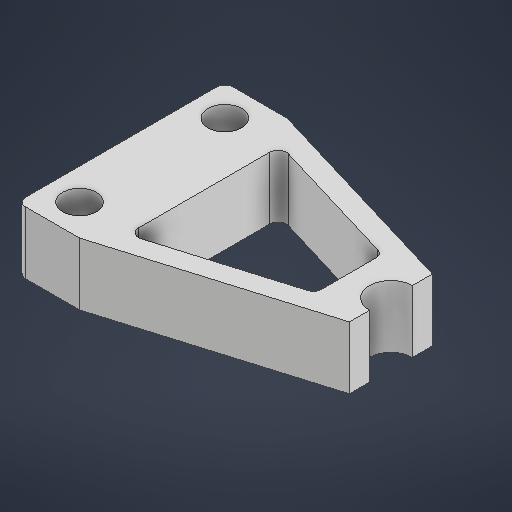
# Autodesk Inventor part: Rod_support_1
Saved by Autodesk Inventor 2026.2 (Build 302298000, 298)
## iProperties
Created: 2025-12-17
Part Number: Rod_support_1
Material: Generic
Document SubType Name: Modeling
Designer: Cobble
Density: 1 g/cm^3
Appearance: Default
Author: Cobble
Autodesk Inventor part; units mm, degrees
ref_plane "YZ Plane" through (0, 0, 0) normal (1, 0, 0) x (0, 1, 0)
ref_plane "XZ Plane" through (0, 0, 0) normal (0, 1, 0) x (-1, 0, 0)
ref_plane "XY Plane" through (0, 0, 0) normal (0, 0, 1) x (1, 0, 0)
sketch "Sketch1" plane through (0, 0, 0) normal (0, 0, 1) x (1, 0, 0)
  arc A0 (0, 5.15) -> (0, -5.15) centre (0, 0) ccw
  line L0 (0, 5.15) -> (0, 10)
  line L1 (0, -5.15) -> (0, -10)
  line L2 (0, 0) -> (-50, 0)
  line L3 (-50, 0) -> (-50, 25)
  line L4 (-50, 0) -> (-50, -25)
  line L5 (-50, -25) -> (0, -10)
  line L6 (-50, 25) -> (0, 10)
  line L7 (-50, 25) -> (-65, 25)
  line L8 (-65, 25) -> (-65, -25)
  line L9 (-65, -25) -> (-50, -25)
  line L10 (-50, 0) -> (-45, 0)
  line L11 (-45, 0) -> (-45, 23.5)
  line L12 (-45, 0) -> (-45, -23.5)
  line L13 (-5.15, 0) -> (-10.15, 0)
  line L14 (-10.15, 0) -> (-10.15, 13.045)
  line L15 (-10.15, 0) -> (-10.15, -13.045)
  line L16 (-45, -23.5) -> (-45, -18.5)
  line L17 (-45, -18.5) -> (-10.15, -8.045)
  line L18 (-45, 23.5) -> (-45, 18.5)
  line L19 (-45, 18.5) -> (-10.15, 8)
  line L20 (-57.5, 25) -> (-57.5, -25)
  line L21 (-65, 0) -> (-50, 0)
  line L22 (-65, 25) -> (-50, 10)
  line L23 (-65, 25) -> (-43.7868, 25) construction
  line L24 (-65, -25) -> (-50, -10)
  line L25 (-65, -25) -> (-43.7868, -25) construction
  circle A1 centre (-57.5, -17.5) radius 4.05
  circle A2 centre (-57.5, 17.5) radius 4.05
  dimension "d0" = 10.3
  dimension "d3" = 50
  dimension "d4" = 25
  dimension "d5" = 25
  dimension "d6" = 15
  dimension "d7" = 50
  dimension "d8" = 90
  dimension "d9" = 5
  dimension "d10" = 5
  dimension "d11" = 5
  dimension "d12" = 5
  dimension "d13" = 45
  dimension "d14" = 45
  dimension "d15" = 8.1
  dimension "d16" = 8.1
  dimension "d26" = 50
  dimension "d27" = 10
  dimension "d28" = 20
  constraints: 52 end point, 15 point on line, 5 midpoint, 4 perpendicular, 4 vertical, 3 centre point, 3 horizontal, 3 point on circle, 2 equal length, 1 coincident, 1 parallel
  measures "d0" diameter of A0
  measures "d3" distance of L2.start L2.end
  measures "d4" distance of L2.end L3.end
  measures "d5" distance of L2.end L4.end
  measures "d6" distance of L3.end L7.end
  measures "d7" distance of L7.end L8.end
  measures "d8" angle of L8 L7
  measures "d9" distance of L2.end L10.end
  measures "d10" distance of L13.start L13.end
  measures "d11" distance of L12.end L16.end
  measures "d12" distance of L11.end L18.end
  measures "d13" angle of L22 L23
  measures "d14" angle of L25 L24
  measures "d15" diameter of A1
  measures "d16" diameter of A2
  measures "d26" distance of L2.end point (0, 0)
  measures "d27" distance of L1.end point (0, 0)
  measures "d28" distance of L0.end L1.end
extrude "Extrusion1" add sketch "Sketch1" along normal blind 15 contours A0 L2 L14 L6 L0 | A0 L1 L5 L15 L2 | L14 L19 L11 L6 | L12 L5 L4 L2 | L2 L3 L6 L11 | L15 L5 L12 L17 | L21 L20 A2 L22 L3 | L4 L24 A1 L20 L21 | L3 L22 A2 L20 L7 | L4 L9 L20 A1 L24 | L21 L8 L22 A2 L20 | L20 A1 L24 L8 L21 | L20 A2 L22 L7 | L9 L24 A1 L20
sketch "Sketch2" plane through (-65, -25, 0) normal (-1, 0, 0) x (0, 0, 1)
  line L0 (0, 50) -> (0, 0) projected
  line L1 (0, 0) -> (15, 0) projected
  line L2 (15, 50) -> (15, 0) projected
  line L3 (0, 50) -> (15, 50) projected
  line L4 (0, 25) -> (15, 25)
  line L5 (7.5, 25) -> (7.5, 17.5)
  line L6 (7.5, 25) -> (7.5, 32.5)
  circle A0 centre (7.5, 32.5) radius 4.05
  circle A1 centre (7.5, 17.5) radius 4.05
  line L7 (7.5, 32.5) -> (11.55, 32.5)
  line L8 (11.55, 32.5) -> (11.55, 17.5)
  line L9 (7.5, 32.5) -> (3.45, 32.5)
  line L10 (3.45, 32.5) -> (3.45, 17.5)
  dimension "d19" = 7.5
  dimension "d20" = 7.5
  dimension "d21" = 8.1
  dimension "d22" = 8.1
  constraints: 14 end point, 4 point on circle, 2 centre point, 2 coincident, 2 midpoint, 2 perpendicular, 2 vertical, 1 horizontal, 1 point on line
  measures "d19" distance of L5.start L5.end
  measures "d20" distance of L5.start L6.end
  measures "d21" diameter of A0
  measures "d22" diameter of A1
extrude "Extrusion2" cut sketch "Sketch2" against normal up to surface (15 mm away) contours L10 A0 L6 L4 | L4 L5 A1 L10 | L6 A0 L8 L4 | L4 L8 A1 L5 | L9 L6 A0 | A0 L7 L9 | A1 | L6 L7 A0
fillet "Fillet1" radius 2 4 edges at (-45, -18.5, 7.5) (-10.15, -8.045, 7.5) (-45, 18.5, 7.5) (-10.15, 8, 7.5)
fillet "Fillet2" radius 2 2 edges at (-65, -25, 7.5) (-65, 25, 7.5)
body "Solid1"
